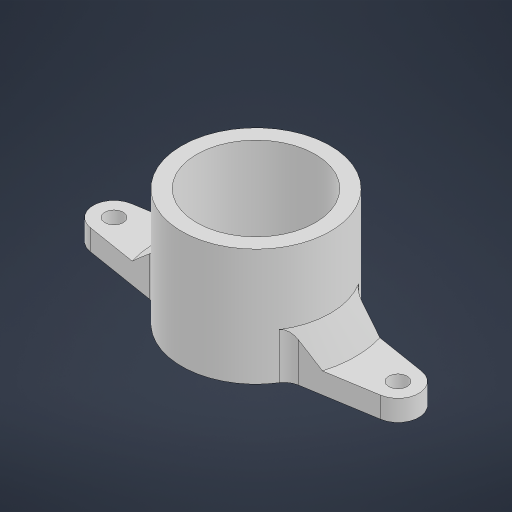
# Autodesk Inventor part: M12Lens_Shutter
Saved by Autodesk Inventor 2024.2 (Build 282272000, 272)
## iProperties
Created: 2024-03-04
Part Number: M12Lens_Shutter
Material: 一般
Document SubType Name: Modeling
Designer: Hanaoka
Density: 1 g/cm^3
Appearance: 既定
Author: Hanaoka
Autodesk Inventor part; units mm, degrees
ref_plane "YZ Plane" through (0, 0, 0) normal (1, 0, 0) x (0, 1, 0)
ref_plane "XZ Plane" through (0, 0, 0) normal (0, 1, 0) x (-1, 0, 0)
ref_plane "XY Plane" through (0, 0, 0) normal (0, 0, 1) x (1, 0, 0)
sketch "スケッチ1" plane through (0, 0, 0) normal (0, 1, 0) x (-1, 0, 0)
  circle A0 centre (0, 0) radius 8.9
  circle A1 centre (0, 0) radius 7.1
  dimension "d0" = 14.2
  dimension "d1" = 17.8
  constraints: 2 centre point, 2 coincident
  measures "d0" diameter of A1
  measures "d1" diameter of A0
extrude "押し出し1" add sketch "スケッチ1" along normal blind 14
sketch "スケッチ2" plane through (0, 0, 0) normal (0, -1, 0) x (1, 0, 0)
  circle A0 centre (-17, 0) radius 1.1
  line L0 (0, -12.46) -> (0, 12.46) construction
  circle A1 centre (17, 0) radius 1.1
  line L1 (-27.3, 0) -> (27.3, 0) construction
  arc A2 (-17.4001, 2.4678) -> (-17.4001, -2.4678) centre (-17, 0) ccw
  line L2 (-17.4001, 2.4678) -> (-7.9505, 4)
  circle A3 centre (0, 0) radius 8.9 projected
  line L3 (-17.4001, -2.4678) -> (-7.9505, -4)
  arc A4 (17.4001, -2.4678) -> (17.4001, 2.4678) centre (17, 0) ccw
  line L4 (17.4001, 2.4678) -> (7.9505, 4)
  line L5 (17.4001, -2.4678) -> (7.9505, -4)
  dimension "d4" = 34
  dimension "d5" = 2.2
  dimension "d6" = 2.5
  dimension "d7" = 8
  constraints: 8 end point, 6 point on circle, 6 symmetric about line, 4 centre point, 2 tangent, 1 coincident, 1 equal length, 1 point on line, 2 other
  measures "d4" distance of A1.centre A0.centre
  measures "d5" diameter of A0
  measures "d6" radius of A2
  measures "d7" distance of L2.end L3.end
extrude "押し出し2" add sketch "スケッチ2" against normal blind 2.5 contours L2 A3 L3 A2 | L4 A4 L5 A3
chamfer "面取り1" distance 3 angle 45 3 edges at (-8.6594, 2.5, 2.0556) (-8.6594, 2.5, -2.0556) (8.9, 2.5, 0)
fillet "フィレット1" radius 2 8 edges at (-7.9505, 4, 4) (-7.9505, 1.25, 4) (-7.9505, 4, -4) (-7.9505, 1.25, -4) (7.9505, 1.25, -4) (7.9505, 4, -4) (7.9505, 1.25, 4) (7.9505, 4, 4)
